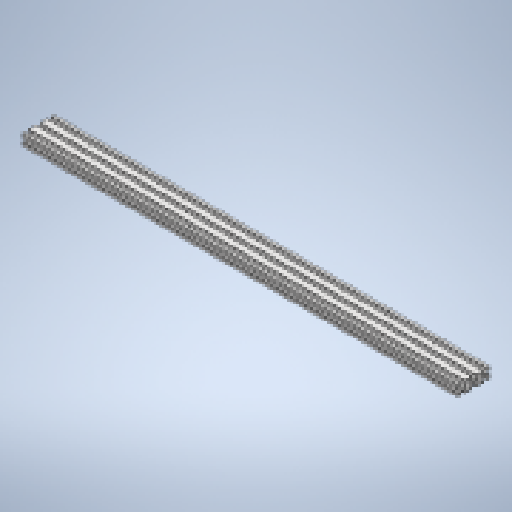
# Autodesk Inventor part: 2030_Extrusion
Saved by Autodesk Inventor 2023 (Build 270158000, 158)
## iProperties
Created: 2022-04-29
Part Number: 2030_Extrusion
Material: Generic
Document SubType Name: Modeling
Designer: plebbb
Density: 1 g/cm^3
Appearance: Default
Author: plebbb
Autodesk Inventor part; units mm, degrees
ref_plane "YZ Plane" through (0, 0, 0) normal (1, 0, 0) x (0, 1, 0)
ref_plane "XZ Plane" through (0, 0, 0) normal (0, 1, 0) x (-1, 0, 0)
ref_plane "XY Plane" through (0, 0, 0) normal (0, 0, 1) x (1, 0, 0)
sketch "Sketch1" plane through (0, 0, 0) normal (1, 0, 0) x (0, 1, 0)
  line L0 (-3.2295, 0) -> (-1.4733, 0)
  line L1 (2.9, 3.8) -> (6.1, 7)
  line L2 (6.1, 7) -> (8.5, 7)
  line L3 (8.5, 7) -> (8.5, 10)
  line L4 (8.5, 10) -> (10, 10)
  line L5 (10, 10) -> (10, 3.7)
  line L6 (10, 3.7) -> (9.25, 3.7)
  line L7 (9.25, 3.7) -> (9.25, 3.2)
  line L8 (9.25, 3.2) -> (8.5, 3.2)
  line L9 (8.5, 3.2) -> (8.5, 5.5)
  line L10 (8.5, 5.5) -> (6.1, 5.5)
  line L11 (6.1, 5.5) -> (3.8, 3.2)
  arc A0 (2.5, 0) -> (0, 2.5) centre (0, 0) ccw
  line L12 (0, 2.5) -> (0, 3.8)
  line L13 (2.5, 0) -> (3.8, 0)
  line L14 (0, 3.8) -> (3.8, 3.8)
  line L15 (3.8, 3.8) -> (3.8, 0)
  point P0 (7.3, 5.5)
  dimension "d1" = 0.5
  dimension "d2" = 10
  dimension "d3" = 5.5
  dimension "d4" = 3.7
  dimension "d5" = 2.5
  dimension "d8" = 10
  dimension "d9" = 1.5
  dimension "d11" = 6.2
  dimension "d12" = 135
  dimension "d13" = 1.5
  constraints: 32 end point, 8 perpendicular, 3 horizontal, 3 vertical alignment, 2 equal length, 2 horizontal alignment, 2 parallel, 2 point on circle, 2 point on line, 1 centre point, 1 coincident, 1 line through centre, 1 midpoint
  measures "d1" distance of L6.end L7.end
  measures "d2" distance from line of point (0, 0) L4
  measures "d3" distance from line of point (0, 0) L10
  measures "d4" distance from line of point (0, 0) L6
  measures "d5" radius of A0
  measures "d8" distance from line of point (0, 0) L5
  measures "d9" distance of L3.end L4.end
  measures "d11" distance between parallel lines of L5 L15
  measures "d12" angle of L15 L11
  measures "d13" distance from line of point (7.3, 5.5) L2
extrude "Extrusion1" add sketch "Sketch1" along normal blind 800
mirror "Mirror1" about plane through (0, 0, 3.8) normal (0, -1, 0)
mirror "Mirror2" about plane through (0, 10, 10) normal (0, 0, 1)
mirror "Mirror3" about plane through (0, -2.5, 0) normal (0, 0, -1)
sketch "Sketch2" plane through (0, 0, 0) normal (-1, 0, 0) x (0, 0, 1)
  arc A0 (20, 2.5) -> (20, -2.5) centre (20, 0) ccw projected
  line L0 (20, 2.5) -> (20, 3.8) projected
  line L1 (20, -2.5) -> (20, -3.8) projected
  line L2 (20, 2.5) -> (20, 3.8) projected
  line L3 (20, 3.8) -> (23.8, 3.8)
  line L4 (20, -3.8) -> (16.8, -3.8) projected
  line L5 (16.2, 2.9) -> (16.2, -2.9) projected
  line L6 (16.2, 0) -> (17.5, 0)
  line L7 (22.5, 0) -> (23.8, 0)
  line L8 (23.2, 3.8) -> (25.5, 6.1)
  line L9 (25.5, 6.1) -> (25.5, 8.5)
  line L10 (25.5, 8.5) -> (23.2, 8.5)
  line L11 (23.2, 8.5) -> (23.2, 9.25)
  line L12 (23.2, 9.25) -> (23.7, 9.25)
  line L13 (23.7, 9.25) -> (23.7, 10)
  line L14 (23.7, 10) -> (29, 10)
  line L15 (30, 9) -> (30, 3.7)
  line L16 (30, 3.7) -> (29.25, 3.7)
  line L17 (29.25, 3.7) -> (29.25, 3.2)
  line L18 (29.25, 3.2) -> (28.5, 3.2)
  line L19 (26.1, 5.5) -> (23.8, 3.2)
  line L20 (26.1, 5.5) -> (28.5, 5.5)
  line L21 (28.5, 5.5) -> (28.5, 3.2)
  arc A1 (22.5, 0) -> (20, 2.5) centre (20, 0) ccw
  line L22 (23.8, 3.8) -> (23.8, 0)
  arc A2 (30, 9) -> (29, 10) centre (29, 9) ccw
  line L23 (14.5, 6.1) -> (14.5, 8.5) projected
  line L24 (16.3, 9.25) -> (16.3, 10) projected
  point P0 (0, 0)
  point P1 (25.5, 7.3)
  point P2 (14.5, 7.3)
  point P3 (23.7, 9.625)
  point P4 (16.8, 3.8)
  dimension "d16" = 135
  dimension "d17" = 90
  dimension "d18" = 0.5
  dimension "d19" = 0.5
  dimension "d20" = 1
  dimension "d21" = 1.5
  dimension "d22" = 10
  dimension "d23" = 11
  dimension "d24" = 7.4
  dimension "d25" = 6.4
  dimension "d26" = 10
  constraints: 36 end point, 9 perpendicular, 7 equal length, 5 point on circle, 4 midpoint, 3 horizontal, 3 vertical, 2 centre point, 2 point on line, 2 tangent, 1 coincident, 1 parallel
  measures "d16" angle of L3 L8
  measures "d18" distance of L11.end L12.end
  measures "d19" vertical distance of L15.end L17.end
  measures "d20" radius of A2
  measures "d21" distance between parallel lines of L14 L10
  measures "d22" distance from line of A0.centre L14
  measures "d23" distance of point (25.5, 7.3) point (14.5, 7.3)
  measures "d24" distance from line of point (23.7, 9.625) L24
  measures "d25" distance of L8.start point (16.8, 3.8)
  measures "d26" distance from line of L15 A0.centre
extrude "Extrusion2" add sketch "Sketch2" against normal blind 800
mirror "Mirror4" about plane through (0, 0, 23.8) normal (0, -1, 0) of "Extrusion2"
mirror "Mirror5" about plane through (0, 0, 0) normal (0, 0, 1) of "Extrusion2", "Mirror4"
body "Solid1"
